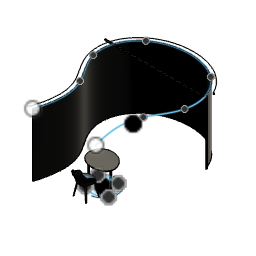
Installation v5 v7 (Autodesk Fusion 360 design; units mm, degrees)
Autodesk Fusion 360 part; units mm, degrees
sketch "Sketch1" plane through (0, 0, 0) normal (0, 0, 1) x (1, 0, 0)
  circle A0 centre (0, 0) radius 450 construction
  spline S0 degree 5 poles (-295.3876, -272.3219) (-273.2624, -287.7834) (-225.7741, -315.9547) (-145.8453, -349.2324) (-27.2342, -373.3808) (124.0079, -367.2514) (260.0357, -325.1509) (364.2834, -250.4054) (424.2227, -149.29) (434.7178, -31.3635) (398.0119, 91.3654) (321.2553, 206.1137) (214.8346, 300.7877) (90.5861, 365.4145) (-40.1286, 393.955) (-167.0688, 384.5566) (-280.9052, 338.8019) (-373.2644, 261.3786) (-436.7484, 159.6194) (-464.8694, 43.3109) (-452.7846, -76.2282) (-409.3132, -165.1441) (-358.5253, -223.186) (-317.5128, -256.8605) (-295.3876, -272.3219) knots 0 0 0 0 0 0 0.05 0.1 0.15 0.2 0.25 0.3 0.35 0.4 0.45 0.5 0.55 0.6 0.65 0.7 0.75 0.8 0.85 0.9 0.95 1 1 1 1 1 1
  line L0 (-334.9887, -121.7814) -> (-304.9887, -121.7814)
  line L1 (-304.9887, -121.7814) -> (-304.9887, -151.7814)
  line L2 (-304.9887, -151.7814) -> (-334.9887, -151.7814)
  line L3 (-334.9887, -151.7814) -> (-334.9887, -121.7814)
  line L4 (-78.7774, 326.9135) -> (-48.7774, 326.9135)
  line L5 (-48.7774, 326.9135) -> (-48.7774, 296.9135)
  line L6 (-78.7774, 296.9135) -> (-78.7774, 326.9135)
  line L7 (-48.7774, 296.9135) -> (-78.7774, 296.9135)
  line L8 (321.7966, -71.0593) -> (351.7966, -71.0593)
  line L9 (351.7966, -71.0593) -> (351.7966, -101.0593)
  line L10 (321.7966, -101.0593) -> (321.7966, -71.0593)
  line L11 (351.7966, -101.0593) -> (321.7966, -101.0593)
  point P0 (384.2782, -203.8544)
  point P1 (163.8461, 322.1769)
  point P2 (-389.3701, 225.5902)
  dimension "d1" = 900
  dimension "d2" = 30
  dimension "d3" = 30
  dimension "d4" = 30
  dimension "d5" = 30
  dimension "d6" = 30
  dimension "d7" = 30
  constraint coincident A0.centre origin
  constraint coincident A0 P2
  constraint horizontal L0
  constraint vertical L1
  constraint horizontal L2
  constraint vertical L3
  constraint horizontal L4
  constraint vertical L5
  constraint horizontal L7
  constraint vertical L6
  constraint horizontal L8
  constraint vertical L9
  constraint horizontal L11
  constraint vertical L10
  measures "d1" diameter of A0
  measures "d2" distance of L0.start L0.end
  measures "d3" distance of L0.start L2.end
  measures "d4" distance of L4.end L4.start
  measures "d5" distance of L6.start L4.start
  measures "d6" distance of L8.end L8.start
  measures "d7" distance of L10.start L8.start
extrude "Extrude1" add sketch "Sketch1" along normal blind 20 from surface at 700 contours S0 | L0 L1 L2 L3 | L4 L5 L6 L7 | L8 L9 L10 L11 makes body 1
extrude "Extrude2" add sketch "Sketch1" along normal blind 690 separate body contours L0 L1 L2 L3 | L4 L5 L6 L7 | L8 L9 L10 L11 makes body 2 at (-68.7774, 326.9135, 460) makes body 3 at (-304.9887, -131.7814, 460) makes body 4 at (331.7966, -71.0593, 460)
other "Base Mesh Feature1"
ref_plane "WorkPlane1" through (0, 0, 2200) normal (0, 0, 1) x (1, 0, 0)
sketch "Sketch2" plane through (0, 0, 2200) normal (0, 0, 1) x (1, 0, 0)
  spline S0 degree 5 poles (-1045.6504, -1181.7815) (-1022.1465, -1106.6212) (-979.9093, -959.7938) (-930.8649, -750.0329) (-894.1347, -491.3415) (-895.3066, -202.3813) (-941.1434, 54.163) (-1026.4556, 282.5499) (-1142.4043, 489.9639) (-1275.1699, 687.7374) (-1407.3014, 889.0674) (-1519.8575, 1105.5498) (-1594.2206, 1344.4204) (-1614.1628, 1604.7463) (-1567.4049, 1876.6066) (-1446.4203, 2144.632) (-1249.5474, 2390.5494) (-981.7927, 2595.9613) (-656.3649, 2745.379) (-293.6428, 2827.685) (82.0692, 2836.1888) (445.091, 2769.0677) (771.2829, 2629.7844) (1040.5882, 2427.3221) (1240.304, 2177.1047) (1365.9652, 1899.4898) (1419.6871, 1615.7629) (1409.2422, 1344.617) (1346.8409, 1098.8434) (1248.1668, 880.8868) (1130.965, 682.7713) (1013.1412, 491.0069) (911.0934, 289.9592) (837.7152, 66.2317) (801.2423, -188.6484) (806.5142, -479.7209) (845.9312, -743.4171) (895.5814, -958.8479) (937.597, -1110.3055) (960.8337, -1187.9936) knots 0 0 0 0 0 0 0.028571 0.057143 0.085714 0.114286 0.142857 0.171429 0.2 0.228571 0.257143 0.285714 0.314286 0.342857 0.371429 0.4 0.428571 0.457143 0.485714 0.514286 0.542857 0.571429 0.6 0.628571 0.657143 0.685714 0.714286 0.742857 0.771429 0.8 0.828571 0.857143 0.885714 0.914286 0.942857 0.971429 1 1 1 1 1 1
  point P0 (-1058.0744, 327.7405)
  point P1 (-1557.927, 1251.0049)
  point P2 (-1117.3026, 2479.7884)
  point P3 (902.4901, 2518.2795)
  point P4 (1371.2944, 1219.975)
  point P5 (942.1976, 340.1646)
sketch "Sketch4" plane through (0, 0, 0) normal (0, 1, 0) x (1, 0, 0)
  circle A0 centre (960.8337, -2200) radius 10
  point P0 (960.8337, -2200)
  dimension "d14" = 20
  constraint coincident P0 A0.centre
  measures "d14" diameter of A0
sweep "Sweep1" add profiles "Sketch4" path "Sketch2" along S0 section 1 separate body makes body 5
sketch "Sketch5" plane through (0, 0, 0) normal (0, 0, 1) x (1, 0, 0)
  line L0 (970.8337, 0) -> (950.8337, 0)
  spline S0 degree 3 poles (950.8337, 0) (943.4447, -36.9767) (937.4196, -75.261) (932.8734, -115.0232) (928.9165, -149.6308) (926.0801, -185.3568) (924.4314, -222.2781) (921.5961, -285.7725) (922.2803, -352.8125) (926.7417, -423.5971) (930.0603, -476.2507) (935.4662, -530.9704) (943.0246, -587.7789) (954.1336, -671.2737) (969.896, -759.2819) (990.4096, -851.7695) (1010.4282, -942.025) (1034.9669, -1036.5413) (1064.0496, -1135.2476) knots 0 0 0 0 0.013927 0.013927 0.013927 0.026048 0.026048 0.026048 0.046893 0.046893 0.046893 0.062398 0.062398 0.062398 0.085188 0.085188 0.085188 0.107428 0.107428 0.107428 0.107428
  line L1 (1064.0496, -1135.2476) -> (1081.8589, -1126.1466)
  spline S1 degree 3 poles (950.8337, 0) (943.4447, -36.9767) (937.4196, -75.261) (932.8734, -115.0232) (928.9165, -149.6308) (926.0801, -185.3568) (924.4314, -222.2781) (921.5961, -285.7725) (922.2803, -352.8125) (926.7417, -423.5971) (930.0603, -476.2507) (935.4662, -530.9704) (943.0246, -587.7789) (954.1336, -671.2737) (969.896, -759.2819) (990.4096, -851.7695) (1010.4282, -942.025) (1034.9669, -1036.5413) (1064.0496, -1135.2476) knots 0 0 0 0 0.013927 0.013927 0.013927 0.026048 0.026048 0.026048 0.046893 0.046893 0.046893 0.062398 0.062398 0.062398 0.085188 0.085188 0.085188 0.107428 0.107428 0.107428 0.107428
  line L2 (970.8337, 0) -> (950.8337, 0)
  spline S2 degree 3 poles (950.8337, 0) (958.7924, 39.8275) (968.3329, 78.1374) (979.3047, 115.2155) (990.0921, 151.6705) (1002.2635, 186.9357) (1015.673, 221.3468) (1028.8571, 255.1795) (1043.2397, 288.1885) (1058.6672, 320.7359) (1073.8354, 352.7363) (1090.0152, 384.2923) (1107.0214, 415.7544) (1123.7419, 446.6877) (1141.2622, 477.5309) (1159.3501, 508.6094) (1177.1342, 539.1657) (1195.4668, 569.95) (1214.0663, 601.2533) (1232.3532, 632.0306) (1250.8973, 663.3101) (1269.3787, 695.3415) (1287.5495, 726.8346) (1305.6588, 759.0552) (1323.3659, 792.2058) (1340.7754, 824.7993) (1357.7951, 858.2927) (1374.0806, 892.8315) (1390.0923, 926.7899) (1405.3931, 961.7598) (1419.6514, 997.819) (1433.67, 1033.2723) (1446.6799, 1069.7789) (1458.3785, 1107.3441) (1469.8806, 1144.278) (1480.1146, 1182.2346) (1488.8182, 1221.155) (1497.3755, 1259.4213) (1504.4532, 1298.6189) (1509.83, 1338.638) (1515.1164, 1377.9846) (1518.7588, 1418.1248) (1520.5741, 1458.9087) (1522.3588, 1499.0072) (1522.3775, 1539.7274) (1520.4804, 1580.8917) (1518.6151, 1621.3642) (1514.8979, 1662.2654) (1509.2086, 1703.3985) (1503.6148, 1743.8404) (1496.1147, 1784.506) (1486.6159, 1825.1863) (1470.4135, 1894.5764) (1448.3831, 1964.0147) (1420.2356, 2032.3494) (1402.5715, 2075.2334) (1382.5026, 2117.6798) (1360.0069, 2159.3868) (1339.1222, 2198.1069) (1316.1461, 2236.1893) (1291.0946, 2273.3899) (1267.1946, 2308.8807) (1241.4055, 2343.5686) (1213.772, 2377.2461) (1187.02, 2409.8494) (1158.5395, 2441.5052) (1128.4001, 2472.0357) (1084.8345, 2516.1668) (1037.7982, 2557.9413) (987.6088, 2596.8889) (930.8772, 2640.9133) (870.1161, 2681.3218) (805.9432, 2717.5939) (739.3151, 2755.2536) (669.0132, 2788.4538) (595.869, 2816.8103) (522.667, 2845.1892) (446.621, 2868.7201) (368.6465, 2887.1828) (291.953, 2905.3422) (213.3953, 2918.6003) (133.8962, 2926.8689) (56.3672, 2934.9325) (-22.0556, 2938.2518) (-100.4891, 2936.8426) (-176.6527, 2935.4743) (-252.8249, 2929.6479) (-328.1946, 2919.4591) (-401.2251, 2909.5866) (-473.5009, 2895.6186) (-544.3017, 2877.711) (-612.8299, 2860.3783) (-679.9753, 2839.355) (-745.116, 2814.8424) (-808.1304, 2791.1299) (-869.2681, 2764.1521) (-928.0059, 2734.1479) (-984.8102, 2705.1314) (-1039.3692, 2673.2842) (-1091.2606, 2638.8815) (-1141.4366, 2605.6161) (-1189.1178, 2569.962) (-1233.9851, 2532.2217) (-1277.3659, 2495.7318) (-1318.1158, 2457.2921) (-1356.0101, 2417.2212) (-1392.6476, 2378.4793) (-1426.6159, 2338.214) (-1457.7763, 2296.743) (-1487.9026, 2256.6482) (-1515.4047, 2215.4272) (-1540.2127, 2173.3808) (-1564.1971, 2132.7302) (-1585.6637, 2091.3086) (-1604.5946, 2049.3914) (-1622.897, 2008.8659) (-1638.8296, 1967.8776) (-1652.4148, 1926.6721) (-1665.549, 1886.8348) (-1676.4893, 1846.7948) (-1685.2894, 1806.7657) (-1693.7973, 1768.0657) (-1700.3049, 1729.3761) (-1704.889, 1690.8773) (-1711.4363, 1635.8901) (-1714.055, 1581.2964) (-1713.0637, 1527.5601) (-1711.9681, 1468.1721) (-1706.4608, 1409.8369) (-1697.1263, 1353.0382) (-1687.6919, 1295.6311) (-1674.349, 1239.7988) (-1657.8627, 1185.8237) (-1641.8433, 1133.3768) (-1622.8605, 1082.6826) (-1601.7209, 1033.7639) (-1581.5675, 987.1273) (-1559.4588, 942.1012) (-1536.1249, 898.5156) (-1514.0928, 857.3616) (-1490.9706, 817.4872) (-1467.3541, 778.6388) (-1445.1658, 742.1398) (-1422.5417, 706.5436) (-1399.9424, 671.5933) (-1378.7647, 638.8418) (-1357.6092, 606.6561) (-1336.8189, 574.8091) (-1317.363, 545.0063) (-1298.2273, 515.4996) (-1279.6565, 486.0994) (-1256.04, 448.7114) (-1233.3417, 411.4951) (-1211.9624, 374.0644) (-1187.065, 330.4744) (-1163.9602, 286.5939) (-1143.08, 241.827) (-1123.4555, 199.7524) (-1105.7888, 156.8923) (-1090.3042, 112.7693) (-1076.2615, 72.7549) (-1064.0098, 31.7016) (-1053.6827, -10.7109) (-1044.4889, -48.4688) (-1036.8199, -87.3041) (-1030.7672, -127.4108) (-1024.4423, -169.3209) (-1019.8826, -212.6204) (-1017.1917, -257.4807) (-1013.9084, -312.2175) (-1013.4093, -369.2815) (-1015.8648, -428.8677) (-1018.7141, -498.0126) (-1025.5452, -570.5542) (-1036.5547, -646.6169) (-1048.1633, -726.8184) (-1064.4175, -810.9298) (-1085.448, -898.9531) (-1105.971, -984.852) (-1131.0394, -1074.4712) (-1160.7111, -1167.7575) knots 0.10742761 0.10742761 0.10742761 0.10742761 0.12242786 0.12242786 0.12242786 0.13717602 0.13717602 0.13717602 0.15167633 0.15167633 0.15167633 0.16593295 0.16593295 0.16593295 0.17994998 0.17994998 0.17994998 0.19373145 0.19373145 0.19373145 0.20728131 0.20728131 0.20728131 0.22060345 0.22060345 0.22060345 0.23370171 0.23370171 0.23370171 0.24657984 0.24657984 0.24657984 0.25924155 0.25924155 0.25924155 0.27169047 0.27169047 0.27169047 0.28393018 0.28393018 0.28393018 0.29596419 0.29596419 0.29596419 0.30779596 0.30779596 0.30779596 0.3194289 0.3194289 0.3194289 0.33086633 0.33086633 0.33086633 0.35037565 0.35037565 0.35037565 0.36261888 0.36261888 0.36261888 0.37398531 0.37398531 0.37398531 0.38482931 0.38482931 0.38482931 0.39532738 0.39532738 0.39532738 0.41050205 0.41050205 0.41050205 0.42765473 0.42765473 0.42765473 0.44546364 0.44546364 0.44546364 0.4632866 0.4632866 0.4632866 0.48081675 0.48081675 0.48081675 0.49791248 0.49791248 0.49791248 0.51451346 0.51451346 0.51451346 0.53059923 0.53059923 0.53059923 0.54616864 0.54616864 0.54616864 0.56122985 0.56122985 0.56122985 0.57579528 0.57579528 0.57579528 0.5898792 0.5898792 0.5898792 0.60349652 0.60349652 0.60349652 0.61666218 0.61666218 0.61666218 0.62939092 0.62939092 0.62939092 0.64169713 0.64169713 0.64169713 0.65359477 0.65359477 0.65359477 0.66509736 0.66509736 0.66509736 0.67621802 0.67621802 0.67621802 0.69210148 0.69210148 0.69210148 0.7096555 0.7096555 0.7096555 0.72739757 0.72739757 0.72739757 0.74463728 0.74463728 0.74463728 0.76107271 0.76107271 0.76107271 0.77659121 0.77659121 0.77659121 0.79117127 0.79117127 0.79117127 0.8048341 0.8048341 0.8048341 0.81761996 0.81761996 0.81761996 0.83387962 0.83387962 0.83387962 0.85281487 0.85281487 0.85281487 0.87061131 0.87061131 0.87061131 0.88675059 0.88675059 0.88675059 0.90111862 0.90111862 0.90111862 0.9161327 0.9161327 0.9161327 0.93445231 0.93445231 0.93445231 0.95571069 0.95571069 0.95571069 0.97812583 0.97812583 0.97812583 1 1 1 1
  line L3 (-1180.5642, -1165.3378) -> (-1160.7111, -1167.7575)
  spline S3 degree 3 poles (950.8337, 0) (958.7924, 39.8275) (968.3329, 78.1374) (979.3047, 115.2155) (990.0921, 151.6705) (1002.2635, 186.9357) (1015.673, 221.3468) (1028.8571, 255.1795) (1043.2397, 288.1885) (1058.6672, 320.7359) (1073.8354, 352.7363) (1090.0152, 384.2923) (1107.0214, 415.7544) (1123.7419, 446.6877) (1141.2622, 477.5309) (1159.3501, 508.6094) (1177.1342, 539.1657) (1195.4668, 569.95) (1214.0663, 601.2533) (1232.3532, 632.0306) (1250.8973, 663.3101) (1269.3787, 695.3415) (1287.5495, 726.8346) (1305.6588, 759.0552) (1323.3659, 792.2058) (1340.7754, 824.7993) (1357.7951, 858.2927) (1374.0806, 892.8315) (1390.0923, 926.7899) (1405.3931, 961.7598) (1419.6514, 997.819) (1433.67, 1033.2723) (1446.6799, 1069.7789) (1458.3785, 1107.3441) (1469.8806, 1144.278) (1480.1146, 1182.2346) (1488.8182, 1221.155) (1497.3755, 1259.4213) (1504.4532, 1298.6189) (1509.83, 1338.638) (1515.1164, 1377.9846) (1518.7588, 1418.1248) (1520.5741, 1458.9087) (1522.3588, 1499.0072) (1522.3775, 1539.7274) (1520.4804, 1580.8917) (1518.6151, 1621.3642) (1514.8979, 1662.2654) (1509.2086, 1703.3985) (1503.6148, 1743.8404) (1496.1147, 1784.506) (1486.6159, 1825.1863) (1470.4135, 1894.5764) (1448.3831, 1964.0147) (1420.2356, 2032.3494) (1402.5715, 2075.2334) (1382.5026, 2117.6798) (1360.0069, 2159.3868) (1339.1222, 2198.1069) (1316.1461, 2236.1893) (1291.0946, 2273.3899) (1267.1946, 2308.8807) (1241.4055, 2343.5686) (1213.772, 2377.2461) (1187.02, 2409.8494) (1158.5395, 2441.5052) (1128.4001, 2472.0357) (1084.8345, 2516.1668) (1037.7982, 2557.9413) (987.6088, 2596.8889) (930.8772, 2640.9133) (870.1161, 2681.3218) (805.9432, 2717.5939) (739.3151, 2755.2536) (669.0132, 2788.4538) (595.869, 2816.8103) (522.667, 2845.1892) (446.621, 2868.7201) (368.6465, 2887.1828) (291.953, 2905.3422) (213.3953, 2918.6003) (133.8962, 2926.8689) (56.3672, 2934.9325) (-22.0556, 2938.2518) (-100.4891, 2936.8426) (-176.6527, 2935.4743) (-252.8249, 2929.6479) (-328.1946, 2919.4591) (-401.2251, 2909.5866) (-473.5009, 2895.6186) (-544.3017, 2877.711) (-612.8299, 2860.3783) (-679.9753, 2839.355) (-745.116, 2814.8424) (-808.1304, 2791.1299) (-869.2681, 2764.1521) (-928.0059, 2734.1479) (-984.8102, 2705.1314) (-1039.3692, 2673.2842) (-1091.2606, 2638.8815) (-1141.4366, 2605.6161) (-1189.1178, 2569.962) (-1233.9851, 2532.2217) (-1277.3659, 2495.7318) (-1318.1158, 2457.2921) (-1356.0101, 2417.2212) (-1392.6476, 2378.4793) (-1426.6159, 2338.214) (-1457.7763, 2296.743) (-1487.9026, 2256.6482) (-1515.4047, 2215.4272) (-1540.2127, 2173.3808) (-1564.1971, 2132.7302) (-1585.6637, 2091.3086) (-1604.5946, 2049.3914) (-1622.897, 2008.8659) (-1638.8296, 1967.8776) (-1652.4148, 1926.6721) (-1665.549, 1886.8348) (-1676.4893, 1846.7948) (-1685.2894, 1806.7657) (-1693.7973, 1768.0657) (-1700.3049, 1729.3761) (-1704.889, 1690.8773) (-1711.4363, 1635.8901) (-1714.055, 1581.2964) (-1713.0637, 1527.5601) (-1711.9681, 1468.1721) (-1706.4608, 1409.8369) (-1697.1263, 1353.0382) (-1687.6919, 1295.6311) (-1674.349, 1239.7988) (-1657.8627, 1185.8237) (-1641.8433, 1133.3768) (-1622.8605, 1082.6826) (-1601.7209, 1033.7639) (-1581.5675, 987.1273) (-1559.4588, 942.1012) (-1536.1249, 898.5156) (-1514.0928, 857.3616) (-1490.9706, 817.4872) (-1467.3541, 778.6388) (-1445.1658, 742.1398) (-1422.5417, 706.5436) (-1399.9424, 671.5933) (-1378.7647, 638.8418) (-1357.6092, 606.6561) (-1336.8189, 574.8091) (-1317.363, 545.0063) (-1298.2273, 515.4996) (-1279.6565, 486.0994) (-1256.04, 448.7114) (-1233.3417, 411.4951) (-1211.9624, 374.0644) (-1187.065, 330.4744) (-1163.9602, 286.5939) (-1143.08, 241.827) (-1123.4555, 199.7524) (-1105.7888, 156.8923) (-1090.3042, 112.7693) (-1076.2615, 72.7549) (-1064.0098, 31.7016) (-1053.6827, -10.7109) (-1044.4889, -48.4688) (-1036.8199, -87.3041) (-1030.7672, -127.4108) (-1024.4423, -169.3209) (-1019.8826, -212.6204) (-1017.1917, -257.4807) (-1013.9084, -312.2175) (-1013.4093, -369.2815) (-1015.8648, -428.8677) (-1018.7141, -498.0126) (-1025.5452, -570.5542) (-1036.5547, -646.6169) (-1048.1633, -726.8184) (-1064.4175, -810.9298) (-1085.448, -898.9531) (-1105.971, -984.852) (-1131.0394, -1074.4712) (-1160.7111, -1167.7575) knots 0.10742761 0.10742761 0.10742761 0.10742761 0.12242786 0.12242786 0.12242786 0.13717602 0.13717602 0.13717602 0.15167633 0.15167633 0.15167633 0.16593295 0.16593295 0.16593295 0.17994998 0.17994998 0.17994998 0.19373145 0.19373145 0.19373145 0.20728131 0.20728131 0.20728131 0.22060345 0.22060345 0.22060345 0.23370171 0.23370171 0.23370171 0.24657984 0.24657984 0.24657984 0.25924155 0.25924155 0.25924155 0.27169047 0.27169047 0.27169047 0.28393018 0.28393018 0.28393018 0.29596419 0.29596419 0.29596419 0.30779596 0.30779596 0.30779596 0.3194289 0.3194289 0.3194289 0.33086633 0.33086633 0.33086633 0.35037565 0.35037565 0.35037565 0.36261888 0.36261888 0.36261888 0.37398531 0.37398531 0.37398531 0.38482931 0.38482931 0.38482931 0.39532738 0.39532738 0.39532738 0.41050205 0.41050205 0.41050205 0.42765473 0.42765473 0.42765473 0.44546364 0.44546364 0.44546364 0.4632866 0.4632866 0.4632866 0.48081675 0.48081675 0.48081675 0.49791248 0.49791248 0.49791248 0.51451346 0.51451346 0.51451346 0.53059923 0.53059923 0.53059923 0.54616864 0.54616864 0.54616864 0.56122985 0.56122985 0.56122985 0.57579528 0.57579528 0.57579528 0.5898792 0.5898792 0.5898792 0.60349652 0.60349652 0.60349652 0.61666218 0.61666218 0.61666218 0.62939092 0.62939092 0.62939092 0.64169713 0.64169713 0.64169713 0.65359477 0.65359477 0.65359477 0.66509736 0.66509736 0.66509736 0.67621802 0.67621802 0.67621802 0.69210148 0.69210148 0.69210148 0.7096555 0.7096555 0.7096555 0.72739757 0.72739757 0.72739757 0.74463728 0.74463728 0.74463728 0.76107271 0.76107271 0.76107271 0.77659121 0.77659121 0.77659121 0.79117127 0.79117127 0.79117127 0.8048341 0.8048341 0.8048341 0.81761996 0.81761996 0.81761996 0.83387962 0.83387962 0.83387962 0.85281487 0.85281487 0.85281487 0.87061131 0.87061131 0.87061131 0.88675059 0.88675059 0.88675059 0.90111862 0.90111862 0.90111862 0.9161327 0.9161327 0.9161327 0.93445231 0.93445231 0.93445231 0.95571069 0.95571069 0.95571069 0.97812583 0.97812583 0.97812583 1 1 1 1
  spline S4 degree 5 poles (-1045.6504, -1181.7815) (-1022.1465, -1106.6212) (-979.9093, -959.7938) (-930.8649, -750.0329) (-894.1347, -491.3415) (-895.3066, -202.3813) (-941.1434, 54.163) (-1026.4556, 282.5499) (-1142.4043, 489.9639) (-1275.1699, 687.7374) (-1407.3014, 889.0674) (-1519.8575, 1105.5498) (-1594.2206, 1344.4204) (-1614.1628, 1604.7463) (-1567.4049, 1876.6066) (-1446.4203, 2144.632) (-1249.5474, 2390.5494) (-981.7927, 2595.9613) (-656.3649, 2745.379) (-293.6428, 2827.685) (82.0692, 2836.1888) (445.091, 2769.0677) (771.2829, 2629.7844) (1040.5882, 2427.3221) (1240.304, 2177.1047) (1365.9652, 1899.4898) (1419.6871, 1615.7629) (1409.2422, 1344.617) (1346.8409, 1098.8434) (1248.1668, 880.8868) (1130.965, 682.7713) (1013.1412, 491.0069) (911.0934, 289.9592) (837.7152, 66.2317) (801.2423, -188.6484) (806.5142, -479.7209) (845.9312, -743.4171) (895.5814, -958.8479) (937.597, -1110.3055) (960.8337, -1187.9936) knots 0 0 0 0 0 0 0.028571 0.057143 0.085714 0.114286 0.142857 0.171429 0.2 0.228571 0.257143 0.285714 0.314286 0.342857 0.371429 0.4 0.428571 0.457143 0.485714 0.514286 0.542857 0.571429 0.6 0.628571 0.657143 0.685714 0.714286 0.742857 0.771429 0.8 0.828571 0.857143 0.885714 0.914286 0.942857 0.971429 1 1 1 1 1 1
  spline S5 degree 3 poles (-1055.1946, -1178.7969) (-1005.6425, -1020.3401) (-968.8799, -871.3132) (-944.8461, -731.7055) (-924.8632, -615.6286) (-913.6903, -506.0733) (-911.0601, -402.8355) (-908.5121, -302.8239) (-913.9905, -208.7513) (-926.8774, -120.0869) (-938.4782, -40.2707) (-956.0824, 35.1643) (-978.8836, 106.9385) (-1000.1716, 173.9492) (-1025.9932, 237.7675) (-1055.3435, 299.2817) (-1085.6666, 362.8349) (-1119.7584, 423.9347) (-1156.0459, 483.9005) (-1199.9225, 556.4073) (-1247.0107, 627.2815) (-1293.7934, 699.1292) (-1333.6676, 760.367) (-1373.2952, 822.3335) (-1410.2757, 886.4403) (-1444.4285, 945.6451) (-1476.3127, 1006.6884) (-1504.0445, 1070.2862) (-1529.2447, 1128.078) (-1551.0101, 1187.982) (-1568.044, 1250.08) (-1584.7666, 1311.0426) (-1596.9248, 1374.1194) (-1603.4798, 1438.9145) (-1610.5253, 1508.5588) (-1611.0911, 1580.1826) (-1604.1943, 1652.7699) (-1597.1334, 1727.084) (-1582.2449, 1802.3977) (-1558.8724, 1877.2313) (-1535.5, 1952.0642) (-1503.6398, 2026.4052) (-1463.1021, 2098.5534) (-1424.0397, 2168.0757) (-1376.9193, 2235.5508) (-1322.0293, 2299.4192) (-1268.5514, 2361.6445) (-1207.6965, 2420.4369) (-1140.2029, 2474.4674) (-1071.5651, 2529.414) (-996.0638, 2579.4302) (-914.9733, 2623.3522) (-828.9526, 2669.9446) (-736.6495, 2709.6746) (-640.0891, 2741.5039) (-538.7307, 2774.9147) (-432.6935, 2799.6156) (-324.6919, 2814.8414) (-215.7283, 2830.2028) (-104.7809, 2835.9162) (5.2028, 2831.6878) (111.1602, 2827.6141) (216.2088, 2814.3139) (317.7916, 2791.9913) (413.7253, 2770.9101) (506.5596, 2741.7843) (594.3658, 2705.1834) (676.7074, 2670.8604) (754.6207, 2629.9642) (826.8215, 2583.3076) (898.3943, 2537.0567) (964.3499, 2485.1484) (1023.8329, 2428.7062) (1085.5326, 2370.1605) (1140.2656, 2306.7438) (1187.5651, 2240.0019) (1238.5395, 2168.0746) (1280.88, 2092.3004) (1314.5754, 2014.7626) (1347.9369, 1937.9931) (1372.8291, 1859.5105) (1389.7323, 1781.2405) (1405.8261, 1706.7183) (1414.6853, 1632.3987) (1417.0737, 1559.6765) (1419.32, 1491.2803) (1415.8477, 1424.3047) (1407.5208, 1359.5507) (1399.3155, 1295.7428) (1386.3996, 1234.0974) (1369.7768, 1174.9105) (1352.5301, 1113.5022) (1331.2965, 1054.7432) (1307.343, 998.3968) (1280.4914, 935.233) (1250.2299, 875.0932) (1218.4375, 816.9572) (1179.6029, 745.944) (1138.5074, 677.9068) (1098.4505, 610.1952) (1063.4571, 551.043) (1029.2657, 492.102) (997.7664, 431.4998) (968.31, 374.8278) (941.2088, 316.6897) (917.6495, 255.7865) (893.3471, 192.9623) (872.8109, 127.192) (856.9399, 57.468) (840.2893, -15.6806) (828.7699, -93.1782) (823.0486, -175.7574) (816.7284, -266.9804) (817.4834, -364.4031) (825.7859, -468.5133) (835.3013, -587.8332) (854.724, -715.927) (884.279, -852.9976) (907.0088, -958.4142) (935.7178, -1069.1256) (970.4143, -1185.128) knots 0 0 0 0 0.03622344 0.03622344 0.03622344 0.06634146 0.06634146 0.06634146 0.09551829 0.09551829 0.09551829 0.12178344 0.12178344 0.12178344 0.14630545 0.14630545 0.14630545 0.17164027 0.17164027 0.17164027 0.20227352 0.20227352 0.20227352 0.22838308 0.22838308 0.22838308 0.25249611 0.25249611 0.25249611 0.27440782 0.27440782 0.27440782 0.29591896 0.29591896 0.29591896 0.31903997 0.31903997 0.31903997 0.342711 0.342711 0.342711 0.36638182 0.36638182 0.36638182 0.38919112 0.38919112 0.38919112 0.4114136 0.4114136 0.4114136 0.43401283 0.43401283 0.43401283 0.45798608 0.45798608 0.45798608 0.48315052 0.48315052 0.48315052 0.50853914 0.50853914 0.50853914 0.53299835 0.53299835 0.53299835 0.55609738 0.55609738 0.55609738 0.57775884 0.57775884 0.57775884 0.5992319 0.5992319 0.5992319 0.62150518 0.62150518 0.62150518 0.64550898 0.64550898 0.64550898 0.66927493 0.66927493 0.66927493 0.69190289 0.69190289 0.69190289 0.71318478 0.71318478 0.71318478 0.7341557 0.7341557 0.7341557 0.7559137 0.7559137 0.7559137 0.78030414 0.78030414 0.78030414 0.8100971 0.8100971 0.8100971 0.83612397 0.83612397 0.83612397 0.8604629 0.8604629 0.8604629 0.88556947 0.88556947 0.88556947 0.91190921 0.91190921 0.91190921 0.94100596 0.94100596 0.94100596 0.97435351 0.97435351 0.97435351 1 1 1 1
  line L4 (960.8337, -1187.9936) -> (970.4143, -1185.128)
  line L5 (-1055.1946, -1178.7969) -> (-1045.6504, -1181.7815)
  dimension "d22" = -10
  constraint coincident S4.end L4.start
  constraint coincident S4.start L5.end
extrude "Extrude3" add sketch "Sketch5" along normal blind 2000 from surface at 200 separate body contours  makes body 6
sketch "Sketch6" plane through (0, 0, 2200) normal (0, 0, 1) x (1, 0, 0)
  line L0 (-1790.5837, 1866.4463) -> (1609.4163, 1866.4463)
  line L1 (1609.4163, 1866.4463) -> (1609.4163, 1836.4463)
  line L2 (1609.4163, 1836.4463) -> (-1790.5837, 1836.4463)
  line L3 (-1790.5837, 1836.4463) -> (-1790.5837, 1866.4463)
  dimension "d26" = 3400
  dimension "d27" = 30
  constraint horizontal L0
  constraint vertical L1
  constraint horizontal L2
  constraint vertical L3
  measures "d26" distance of L0.start L0.end
  measures "d27" distance of L0.end L1.end
extrude "Extrude4" add sketch "Sketch6" along normal blind 30 separate body makes body 7
